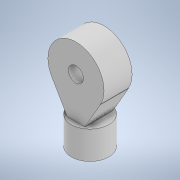
# Autodesk Inventor part: Load Notch Insert
Saved by Autodesk Inventor 2020 (Build 240168000, 168)
## iProperties
Created: 2021-01-30
Part Number: Load Notch Insert
Material: Generic
Document SubType Name: Modeling
Designer: magda
Density: 1 g/cm^3
Appearance: Default
Author: magda
Autodesk Inventor part; units mm, degrees
ref_plane "YZ Plane" through (0, 0, 0) normal (1, 0, 0) x (0, 1, 0)
ref_plane "XZ Plane" through (0, 0, 0) normal (0, 1, 0) x (-1, 0, 0)
ref_plane "XY Plane" through (0, 0, 0) normal (0, 0, 1) x (1, 0, 0)
sketch "Sketch1" plane through (0, 0, 0) normal (0, 0, 1) x (1, 0, 0)
  arc A0 (16.5296, -9.4696) -> (-16.4657, -9.5803) centre (0, 0) ccw
  circle A1 centre (0, 0) radius 5.08
  line L0 (16.5296, -9.4696) -> (16.6574, -9.4696)
  line L1 (16.6574, -9.4696) -> (5.9637, -27.9917)
  line L2 (-5.8359, -27.9917) -> (-16.5296, -9.4696)
  line L3 (-5.8359, -27.9917) -> (5.9637, -27.9917)
  point P0 (0.0639, -19.0499)
  dimension "d0" = 38.1
  dimension "d1" = 10.16
  constraints: 8 end point, 4 point on circle, 2 centre point, 2 coincident, 2 horizontal, 1 point on line, 5 other
  measures "d0" diameter of A0
  measures "d1" diameter of A1
extrude "Extrusion1" add sketch "Sketch1" along normal blind 19.05
sketch "Sketch2" plane through (-5.8359, -27.9917, 0) normal (0, -1, 0) x (1, 0, 0)
  circle A0 centre (5.8941, 9.525) radius 12.7
  line L0 (11.7996, 0) -> (11.7996, 19.05) projected
  line L1 (0, 0) -> (11.7996, 0) projected
  point P0 (5.8359, 0)
  dimension "d4" = 25.4
  dimension "d5" = 5.9055
  dimension "d6" = 9.525
  constraints: 1 centre point
  measures "d4" diameter of A0
  measures "d5" distance from line of A0.centre L0
  measures "d6" distance from line of L1 A0.centre
extrude "Extrusion2" add sketch "Sketch2" along normal blind 19.05
body "Solid1"
